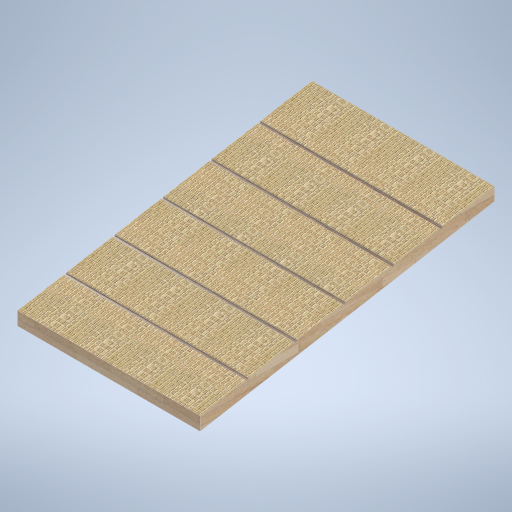
# Autodesk Inventor part: eave_panel_01
Saved by Autodesk Inventor 2024.2 (Build 282272000, 272)
## iProperties
Created: 2024-05-23
Part Number: eave_panel_01
Material: Wood (Maple)
Document SubType Name: Modeling
Designer: LOSTER_1
Density: 0.67 g/cm^3
Appearance: Natural Maple - Glossy Dark Tint
Author: LOSTER_1
Autodesk Inventor part; units mm, degrees
ref_plane "YZ Plane" through (0, 0, 0) normal (1, 0, 0) x (0, 1, 0)
ref_plane "XZ Plane" through (0, 0, 0) normal (0, 1, 0) x (-1, 0, 0)
ref_plane "Work Plane2" through (0, 0, 2209) normal (0, 0, 1) x (1, 0, 0)
ref_plane "Work Plane1" through (0, 0, 0) normal (0, 0, 1) x (1, 0, 0)
sketch "Sketch1" plane through (0, 0, 0) normal (0, 0, 1) x (1, 0, 0)
  line L0 (0, 0) -> (1369, 0)
  line L1 (1369, 0) -> (1369, -100)
  line L2 (1369, -100) -> (0, -100)
  line L3 (0, -100) -> (0, 0)
  dimension "d2" = 1369
  dimension "d3" = 100
  constraints: 8 end point, 2 parallel, 1 horizontal, 1 perpendicular
  measures "d2" distance of L1.end L2.end
  measures "d3" distance of L0.end L1.end
sketch "Sketch2" plane through (0, 0, 2209) normal (0, 0, 1) x (1, 0, 0)
  line L0 (0, -100) -> (0, 0) projected
  line L1 (1369, 0) -> (1369, -100) projected
ref_plane "Work Plane3" through (0, -100, 0) normal (1, 0, 0) x (0, 1, 0)
sketch "Sketch3" plane through (0, -100, 0) normal (1, 0, 0) x (0, 1, 0)
  line L0 (0, 2209) -> (100, 2209) projected
  line L1 (0, 0) -> (100, 0) construction
  line L2 (100, 0) -> (-289.5063, 2209)
  line L3 (100, 0) -> (2343.0774, 0) construction
  line L4 (-289.5063, 2209) -> (-389.5063, 2209)
  line L5 (-389.5063, 2209) -> (0, 0)
  dimension "d4" = 100
  dimension "d5" = 100
  constraints: 8 end point, 2 horizontal, 1 equal length
  measures "d4" angle of L3 L2
  measures "d5" distance of L2.end L4.end
sketch "Sketch4" plane through (0, 0, 2209) normal (0, 0, 1) x (1, 0, 0)
  line L0 (0, -389.5063) -> (0, -489.5063) projected
  line L1 (1369, 0) -> (1369, -100) projected
  line L2 (0, -389.5063) -> (1369, -389.5063)
  line L3 (1369, -389.5063) -> (1369, -489.5063)
  line L4 (1369, -489.5063) -> (0, -489.5063)
  line L5 (0, -489.5063) -> (0, -389.5063)
  point P0 (0, 0)
  constraints: 8 end point, 2 parallel, 1 horizontal, 1 perpendicular
loft "Loft1" add profiles "Sketch1", "Sketch4"
sketch "Sketch5" plane through (1369, -100, 0) normal (1, 0, 0) x (0, 0, -1)
  line L0 (0, 100) -> (0, 0) projected
  line L1 (0, 100) -> (-2209, -289.5063) projected
  line L2 (-2209, -289.5063) -> (-2209, -389.5063) projected
  line L3 (0, 0) -> (-2209, -389.5063) projected
  line L4 (-2209, -289.5063) -> (-1864.3173, -228.7294)
  line L5 (0, 100) -> (-2209, -289.5063) projected
  line L6 (-1864.3173, -228.7294) -> (-1864.3173, -238.7294)
  line L7 (-1864.3173, -238.7294) -> (-1844.6211, -235.2565)
  line L8 (-1844.6211, -235.2565) -> (-1844.6211, -225.2565)
  line L9 (-1844.6211, -225.2565) -> (-1499.9384, -164.4796)
  line L10 (-1499.9384, -164.4796) -> (-1499.9384, -174.4796)
  line L11 (-1499.9384, -174.4796) -> (-1480.2423, -171.0066)
  line L12 (-1480.2423, -171.0066) -> (-1480.2423, -161.0066)
  line L13 (-1480.2423, -161.0066) -> (-1135.5595, -100.2298)
  line L14 (-1135.5595, -100.2298) -> (-1135.5595, -110.2298)
  line L15 (-1135.5595, -110.2298) -> (-1116.23, -106.8215)
  line L16 (-1116.23, -106.8215) -> (-1116.23, -96.8215)
  line L17 (-1116.23, -96.8215) -> (-771.5473, -36.0446)
  line L18 (-771.5473, -36.0446) -> (-771.5473, -46.0446)
  line L19 (-771.5473, -46.0446) -> (-752.0292, -42.603)
  line L20 (-752.0292, -42.603) -> (-752.0292, -32.603)
  line L21 (-752.0292, -32.603) -> (-407.3465, 28.1738)
  line L22 (-407.3465, 28.1738) -> (-407.3465, 18.1738)
  line L23 (-407.3465, 18.1738) -> (-387.7831, 21.6234)
  line L24 (-387.7831, 21.6234) -> (-387.7831, 31.6234)
  line L25 (-387.7831, 31.6234) -> (0, 100)
  line L26 (-387.7831, 31.6234) -> (-1864.3173, -228.7294)
  point P0 (-771.5473, -36.0446)
  point P1 (-1135.5595, -100.2298)
  dimension "d10" = 350
  dimension "d11" = 10
  dimension "d12" = 20
  dimension "d13" = 350
  dimension "d14" = 20
  dimension "d15" = 350
  dimension "d16" = 350
  dimension "d17" = 350
  constraints: 44 end point, 8 parallel, 4 point on line, 3 vertical, 1 collinear, 12 other
  measures "d10" distance of L1.end L4.end
  measures "d11" distance of L4.end L6.end
  measures "d12" distance of L6.end L7.end
  measures "d13" distance of L8.end L9.end
  measures "d14" distance of L10.end L11.end
  measures "d15" distance of L12.end L13.end
  measures "d16" distance of L16.end L17.end
  measures "d17" distance of L20.end L21.end
extrude "Extrusion1" cut sketch "Sketch5" against normal through all contours L24 L23 L22 L1 | L20 L19 L18 L1 | L1 L8 L7 L6 | L16 L15 L14 L1 | L1 L12 L11 L10
body "Solid1"
